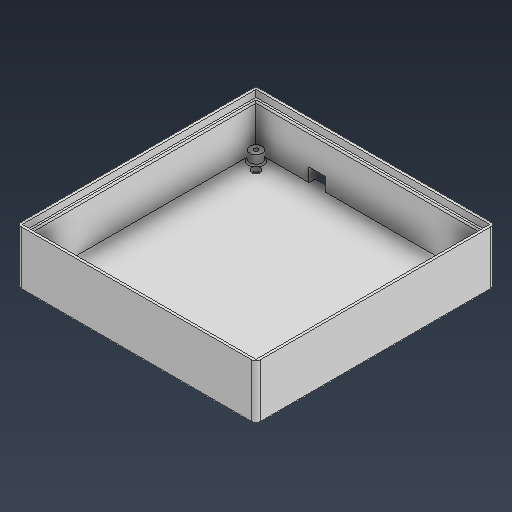
# Autodesk Inventor part: Box
Saved by Autodesk Inventor 2025.3 (Build 293356000, 356)
## iProperties
Created: 2025-09-15
Part Number: Box
Material: Generic
Document SubType Name: Modeling
Designer: tolga
Density: 1 g/cm^3
Appearance: Default
Author: tolga
Autodesk Inventor part; units mm, degrees
ref_plane "YZ Plane" through (0, 0, 0) normal (1, 0, 0) x (0, 1, 0)
ref_plane "XZ Plane" through (0, 0, 0) normal (0, 1, 0) x (-1, 0, 0)
ref_plane "XY Plane" through (0, 0, 0) normal (0, 0, 1) x (1, 0, 0)
sketch "Sketch1" plane through (0, 0, 0) normal (0, 1, 0) x (-1, 0, 0)
  line L0 (0, 0) -> (175, 0)
  line L1 (175, 0) -> (175, -175)
  line L2 (175, -175) -> (0, -175)
  line L3 (0, -175) -> (0, 0)
  dimension "d0" = 175
  dimension "d1" = 175
  constraints: 8 end point, 2 parallel, 1 horizontal, 1 perpendicular
  measures "d0" distance of L1.end L2.end
  measures "d1" distance of L0.end L1.end
extrude "Extrusion1" add sketch "Sketch1" along normal blind 3
sketch "Sketch2" plane through (0, 3, 0) normal (0, 1, 0) x (1, 0, 0)
  line L0 (0, 175) -> (-175, 175) projected
  line L1 (-175, 175) -> (-175, 0) projected
  line L2 (-175, 0) -> (0, 0) projected
  line L3 (0, 0) -> (0, 175) projected
  line L4 (-4.5, 170.5) -> (-170.5, 170.5)
  line L5 (-170.5, 170.5) -> (-170.5, 4.5)
  line L6 (-170.5, 4.5) -> (-4.5, 4.5)
  line L7 (-4.5, 4.5) -> (-4.5, 170.5)
  dimension "d21" = 166
  constraints: 8 end point, 3 other
  measures "d21" distance of L4.start L4.end
extrude "Extrusion2" add sketch "Sketch2" along normal blind 37.09
sketch "Sketch3" plane through (0, 40.09, 0) normal (0, 1, 0) x (1, 0, 0)
  line L0 (-175, 175) -> (-175, 0) projected
  line L1 (-175, 0) -> (0, 0) projected
  line L2 (0, 0) -> (0, 175) projected
  line L3 (0, 175) -> (-175, 175) projected
  line L4 (-4.5, 170.5) -> (-4.5, 4.5) projected
  line L5 (-4.5, 4.5) -> (-170.5, 4.5) projected
  line L6 (-170.5, 4.5) -> (-170.5, 170.5) projected
  line L7 (-170.5, 170.5) -> (-4.5, 170.5) projected
  line L8 (-1.9, 1.9) -> (-1.9, 173.1)
  line L9 (-1.9, 173.1) -> (-173.1, 173.1)
  line L10 (-173.1, 173.1) -> (-173.1, 1.9)
  line L11 (-173.1, 1.9) -> (-1.9, 1.9)
  dimension "d20" = 171.2
  constraints: 8 end point, 3 other
  measures "d20" distance between parallel lines of L11 L9
extrude "Extrusion3" cut sketch "Sketch3" against normal blind 5 contours L11 L10 L9 L8
sketch "Sketch5" plane through (0, 3, 0) normal (0, 1, 0) x (1, 0, 0)
  line L0 (-4.5, 170.5) -> (-170.5, 170.5) construction
  line L1 (-170.5, 170.5) -> (-170.5, 4.5) construction
  line L2 (-170.5, 4.5) -> (-4.5, 4.5) construction
  line L3 (-4.5, 4.5) -> (-4.5, 170.5) construction
  line L4 (-170, 170) -> (-5, 170) construction
  line L5 (-5, 170) -> (-5, 5) construction
  line L6 (-5, 5) -> (-170, 5) construction
  line L7 (-170, 5) -> (-170, 170) construction
  circle A0 centre (-165, 165) radius 4.6
  circle A1 centre (-10, 165) radius 4.6
  circle A2 centre (-165, 10) radius 4.6
  circle A3 centre (-32, 13) radius 4.6
  point P0 (0, 0)
  dimension "d22" = 165
  dimension "d23" = 5
  dimension "d27" = 5
  dimension "d34" = 8
  dimension "d35" = 27
  dimension "d36" = 5
  dimension "d37" = 5
  dimension "d38" = 5
  dimension "d39" = 5
  dimension "d45" = 9.2
  dimension "d46" = 9.2
  dimension "d47" = 9.2
  dimension "d48" = 9.2
  constraints: 8 end point, 4 centre point, 3 other
  measures "d22" distance of L4.start L4.end
  measures "d23" distance from line of L4 A0.centre
  measures "d27" distance from line of L7 A0.centre
  measures "d34" distance from line of L6 A3.centre
  measures "d35" distance from line of L5 A3.centre
  measures "d36" distance from line of L7 A2.centre
  measures "d37" distance from line of L6 A2.centre
  measures "d38" distance from line of L4 A1.centre
  measures "d39" distance from line of L5 A1.centre
  measures "d45" diameter of A2
  measures "d46" diameter of A3
  measures "d47" diameter of A0
  measures "d48" diameter of A1
extrude "Extrusion5" add sketch "Sketch5" along normal blind 7
sketch "Sketch8" plane through (-165, 10, -165) normal (0, 1, 0) x (1, 0, 0)
  circle A0 centre (155, 0) radius 4.6 construction
  circle A1 centre (0, -155) radius 4.6 construction
  circle A2 centre (133, -152) radius 4.6 projected
  circle A3 centre (0, 0) radius 4.6 projected
  point P0 (165, -165)
hole "Hole1" at (-10, 10, -165) at (-165, 10, -10) at (-165, 10, -165) at (-32, 10, -13) direction (0, -1, 0) diameter 3.2 depth 10 tip angle 118
sketch "Sketch9" plane through (0, 0, -175) normal (0, 0, -1) x (-1, 0, 0)
  line L0 (4.5, 35.09) -> (170.5, 35.09) construction
  line L1 (170.5, 3) -> (170.5, 35.09) construction
  line L2 (4.5, 3) -> (170.5, 3) construction
  line L3 (4.5, 3) -> (4.5, 35.09) construction
  line L4 (119.735, 13) -> (131.735, 13)
  line L5 (131.735, 13) -> (131.735, 3)
  line L6 (131.735, 3) -> (119.735, 3)
  line L7 (119.735, 3) -> (119.735, 13)
  line L8 (169.6, 10) -> (160.4, 10) construction
  line L9 (170.5, 11.6) -> (4.5, 11.6) construction
  line L10 (4.5, 3) -> (4.5, 35.09) construction
  point P0 (0, 0)
  point P1 (125.735, 13)
  point P2 (125.735, 3)
  dimension "d58" = 44.765
  dimension "d59" = 12
  dimension "d60" = 10
  dimension "d61" = 1.6
  constraints: 10 end point, 3 perpendicular, 3 point on line, 2 midpoint, 2 parallel, 1 horizontal
  measures "d58" distance from line of L1 point (125.735, 13)
  measures "d59" distance of L5.end L6.end
  measures "d60" distance of L4.end L5.end
  measures "d61" distance between parallel lines of L8 L9
extrude "Extrusion7" cut sketch "Sketch9" against normal up to surface (4.5 mm away)
sketch "Sketch10" plane through (0, 0, 0) normal (0, -1, 0) x (1, 0, 0)
  line L0 (0, 0) -> (0, -175) construction
  line L1 (-175, 0) -> (0, 0) construction
  line L2 (-175, -175) -> (-175, 0) construction
  line L3 (0, -175) -> (-175, -175) construction
  circle A0 centre (-159, -16) radius 3.2
  circle A1 centre (-16, -16) radius 3.2
  circle A2 centre (-159, -159) radius 3.2
  circle A3 centre (-16, -159) radius 3.2
  dimension "d64" = 6.4
  dimension "d65" = 16
  dimension "d66" = 16
  dimension "d69" = 143
  dimension "d72" = 143
  constraints: 4 centre point, 1 horizontal, 1 vertical, 6 other
  measures "d64" diameter of A0
  measures "d65" distance from line of L1 A0.centre
  measures "d66" distance from line of L2 A0.centre
  measures "d69" distance of A0.centre A1.centre
  measures "d72" distance of A0.centre A2.centre
extrude "Extrusion8" cut sketch "Sketch10" against normal up to surface (3 mm away)
sketch "Sketch11" plane through (0, 0, 0) normal (0, -1, 0) x (1, 0, 0)
  circle A0 centre (-16, -16) radius 3.2 projected
  circle A1 centre (-159, -16) radius 3.2 projected
  circle A2 centre (-16, -159) radius 3.2 projected
  circle A3 centre (-159, -159) radius 3.2 projected
  circle A4 centre (-32, -13) radius 1.6 projected
  circle A5 centre (-165, -165) radius 1.6 projected
  circle A6 centre (-165, -10) radius 1.6 projected
  circle A7 centre (-10, -165) radius 1.6 projected
  line L0 (0, -175) -> (-175, -175) projected
  line L1 (0, 0) -> (0, -175) projected
  line L2 (-175, 0) -> (0, 0) projected
  line L3 (-175, -175) -> (-175, 0) projected
  circle A8 centre (-10, -165) radius 3
  circle A9 centre (-165, -165) radius 3
  circle A10 centre (-165, -10) radius 3
  circle A11 centre (-32, -13) radius 3
  dimension "d77" = 6
  dimension "d78" = 6
  dimension "d79" = 6
  dimension "d80" = 6
  constraints: 4 centre point, 4 coincident
  measures "d77" diameter of A8
  measures "d78" diameter of A9
  measures "d79" diameter of A10
  measures "d80" diameter of A11
extrude "Extrusion9" cut sketch "Sketch11" against normal blind 4 contours A8 | A9 | A10 | A11
fillet "Fillet1" radius 3 4 edges at (0, 20.045, -175) (0, 20.045, 0) (-175, 20.045, 0) (-175, 20.045, -175)
fillet "Fillet2" radius 1 8 edges at (-0.8787, 0, -0.8787) (0, 0, -87.5) (-0.8787, 0, -174.1213) (-87.5, 0, -175) (-174.1213, 0, -174.1213) (-175, 0, -87.5) (-174.1213, 0, -0.8787) (-87.5, 0, 0)
fillet "Fillet3" radius 1.1 4 edges at (-170.5, 35.09, -87.5) (-87.5, 35.09, -170.5) (-4.5, 35.09, -87.5) (-87.5, 35.09, -4.5)
fillet "Fillet4" radius 1 4 edges at (-169.6, 3, -10) (-169.6, 3, -165) (-14.6, 3, -165) (-36.6, 3, -13)
equation "\"d27\" = d23"
equation "\"d46\" = d45"
equation "\"d78\" = d77"
equation "\"d79\" = d77"
equation "\"d80\" = d77"
body "Solid1"
